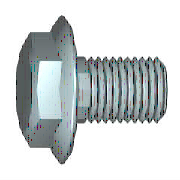
# Autodesk Inventor part: 1_4-20 UNC x 0.625
Saved by Autodesk Inventor 2025.3 (Build 293356030, 356C)
## iProperties
Created: 2024-01-20
Part Number: 1_4-20 UNC x 0.625
Material: Steel, Mild
Description: 1/4"-20 X 5/8" Long Flange Bolt
Document SubType Name: Modeling
Standard: IFI 111
Designer: josh
Standard Revision: 2002
Standards Organization: ANSI
Language: en-US
Size Designation: 1/4-20 UNC x 0.625
Categories: <MemberInstance><Categories><Category DisplayName="Fasteners" InternalName="e4da775c-781d-43d5-af7c-5136215cf5a6" Mnemonic="FSTN"><Category DisplayName="Bolts" InternalName="536e6df0-f778-49ac-b2f2-25c71d2aa0b2" Mnemonic="SCRW"><CategoryParameter DisplayName="Nominal Diameter Designation" InternalName="03caf894-eafd-4c09-a035-916ac084b87b" Mnemonic="nomdiadesig"/><CategoryParameter DisplayName="Nominal Length" InternalName="238ecbaf-3e6c-45dd-aa95-4068c8e0fd02" Mnemonic="nomlen"/><CategoryParameter DisplayName="Thread Designation" InternalName="586d5e89-370a-4089-914f-0110033585c7" Mnemonic="thrdesign"/><CategoryParameter DisplayName="Thread Series Designation" InternalName="87c5849c-b3a5-4c3e-9c9b-2feecef9be86" Mnemonic="thrserdsgn"/><CategoryParameter DisplayName="Nominal Diameter" InternalName="8bbe3f8e-44cf-40a9-a251-3a6edc8168d6" Mnemonic="nomdia"/><CategoryParameter DisplayName="Thread Type" InternalName="b4bbb7bc-d6aa-4c9f-a9a9-4152b9f6fe49" Mnemonic="thrtype"/><CategoryParameter DisplayName="Thread Pitch" InternalName="bb82302e-82d8-4176-8fc1-c5d7bb17d5ad" Mnemonic="pitch1"/><CategoryParameter DisplayName="Threads per Unit" InternalName="bdc6e7d2-ffd0-4d9c-a173-16b95ebb912d" Mnemonic="thrperunit1"/><CategoryParameter DisplayName="Thread Class" InternalName="ebc0d23b-2cc6-4d2a-b376-d52aae53bab6" Mnemonic="thrclss"/><Category DisplayName="Hex Head - Flanged" InternalName="7925b6b6-1575-406f-8bfa-fe006e82b7bc" Mnemonic="FGPLSCREW"><CategoryParameter DisplayName="Width Across Flats" InternalName="448f2cb5-f593-46ea-8e76-5090215a815d" Mnemonic="waflat"/><CategoryParameter DisplayName="Head Height" InternalName="5df4f2f2-b824-4910-9115-49166ccd53b4" Mnemonic="headh"/><CategoryParameter DisplayName="Shank Diameter" InternalName="6799ed14-8456-4cfb-bc01-ee9ecb2cdc2b" Mnemonic="grpdia"/><CategoryParameter DisplayName="Width Across Corners" InternalName="6c4712eb-409b-4c09-a24f-32eb670e2942" Mnemonic="wacor"/><CategoryParameter DisplayName="Type" InternalName="851a99d2-714c-4be1-b4b1-e391fdc059ef" Mnemonic="type"/><CategoryParameter DisplayName="Grip Length" InternalName="a82b65ac-2d41-4fd1-ba9a-aaa8c8b996d2" Mnemonic="grplen"/><CategoryParameter DisplayName="Thread Length" InternalName="f423544c-1850-46c6-9c68-3a3846636699" Mnemonic="thrlen"/></Category></Category></Category><Category DisplayName="DataType" InternalName="23b78d0f-2648-40c6-8793-ca6db495c9e8" Mnemonic="DATATYPE"><CategoryParameter DisplayName="DisplayName" InternalName="05415f3d-3907-474b-a020-eb9d644f4cf3" Mnemonic="DISPLAYNAME"/><CategoryParameter DisplayName="Standard" InternalName="0c0a119c-1e12-4c84-803f-101930972f5e" Mnemonic="STANDARD"/><CategoryParameter DisplayName="Description" InternalName="13903e3d-64b1-4950-80da-f627842ea37f" Mnemonic="DESCRIPTION"/><CategoryParameter DisplayName="Designation" InternalName="2675968c-4ce5-49e0-a4f5-552d29089031" Mnemonic="DESIGNATION"/><CategoryParameter DisplayName="Default Row" InternalName="2af9ec52-faaa-4026-b378-f9fa4afca842" Mnemonic="DEFAULTROW"/><CategoryParameter DisplayName="Folder Name" InternalName="3f06958e-8713-4116-9be7-ed6184ecc97b" Mnemonic="FOLDERNAME"/><CategoryParameter DisplayName="Revision Guid" InternalName="45a75005-10b1-4dfc-8d6d-dfe629f0b93c" Mnemonic="REVISIONGUID"/><CategoryParameter DisplayName="FileName" InternalName="8b46a4cc-9585-4fed-90c3-899f57e09a73" Mnemonic="FILENAME"/><CategoryParameter DisplayName="StdsOrg" InternalName="8f5914e1-4693-403f-8ab5-d37768198c9d" Mnemonic="STDSORG"/><CategoryParameter DisplayName="Family Version" InternalName="914462f6-6e19-4b14-ba84-155b9680b1d0" Mnemonic="FAMILYREVISION"/><CategoryParameter DisplayName="Standard Revision" InternalName="91d5a463-65c2-4fde-b823-3b7fea5e8e17" Mnemonic="STANDARDREVISION"/><CategoryParameter DisplayName="Member Revision" InternalName="a65d44b9-392f-4f4f-857b-e4b3d54996fe" Mnemonic="MEMBERREVISION"/><CategoryParameter DisplayName="ClipFormat" InternalName="bc51e27b-3422-4e78-93ef-cec197ddf230" Mnemonic="CLIPFORMAT"/><CategoryParameter DisplayName="Manufacturer" InternalName="cd6c7a72-a28a-4e50-99a9-2c7f4e13e5ad" Mnemonic="MANUFACTURER"/><CategoryParameter DisplayName="InternalName" InternalName="cf1d0246-76d9-4b4a-8305-fa0409afb5c1" Mnemonic="INTERNALNAME"/><CategoryParameter DisplayName="IsMetric" InternalName="e2385c5b-1ea4-4823-96a8-8de651266ec3" Mnemonic="ISMETRIC"/><Category DisplayName="Part" InternalName="c0e0b642-3bcb-4cc8-9e80-f96d35c4afa4" Mnemonic="PART"><CategoryParameter DisplayName="Part Number" InternalName="016b6077-bfbe-49bd-92c9-d8d59c39c941" Mnemonic="PARTNUMBER"/><CategoryParameter DisplayName="Stock Number" InternalName="4dba7c1c-e26c-444e-836c-b08b433409a8" Mnemonic="STOCKNUMBER"/><CategoryParameter DisplayName="Material Key" InternalName="5c9a8adb-dd2b-4535-b97f-0a94a95fe41f" Mnemonic="MATERIALKEY"/><CategoryParameter DisplayName="Material" InternalName="818a152a-d3c3-49ca-80ee-df7d91421b8e" Mnemonic="MATERIAL"/></Category></Category><Category DisplayName="LegacyMap" InternalName="cd87c42b-3e48-431e-b5c0-1cbeb14dfe77" Mnemonic="LEGACYMAP"><CategoryParameter DisplayName="unique DA member ID" InternalName="0918ad47-427f-4fed-ae26-24c81c58f590" Mnemonic="DACOOKIE"/><CategoryParameter DisplayName="Merge11 ID" InternalName="0ee8fb18-e2ed-4f39-96f6-1f4b5f50aa71" Mnemonic="MERGE11"/><CategoryParameter DisplayName="unique CC member ID" InternalName="5193edd4-b2b0-4ab4-9d54-de900eee34e0" Mnemonic="CCCOOKIE"/><CategoryParameter DisplayName="Split ID" InternalName="72b5c83c-be7f-45c4-ae51-9160ea6deb26" Mnemonic="SPLIT"/><CategoryParameter DisplayName="MemberID" InternalName="8e5e0294-fc51-4c8f-b3d7-003dc5ed94f6" Mnemonic="MEMBERID"/><CategoryParameter DisplayName="CatalogName" InternalName="d99d1e27-aa94-4de2-af4c-c348882a6f4f" Mnemonic="CATALOGNAME"/><CategoryParameter DisplayName="FamilyNumber" InternalName="e705e1f4-09cb-413e-91f9-551b4188271e" Mnemonic="FAMILYNUMBER"/></Category></Categories><FamilyTemplate Id="no0169"><FamilyTemplateParameters><FamilyTemplateParameter ObjectType="kUserParameterObject" ValueType="xs:double" Id="1" ObjectReferenceKey="GUL"/><FamilyTemplateParameter ObjectType="kUserParameterObject" ValueType="xs:double" Id="2" ObjectReferenceKey="SPD"/><FamilyTemplateParameter ObjectType="kUserParameterObject" ValueType="xs:double" Id="3" ObjectReferenceKey="TPU"/><FamilyTemplateParameter ObjectType="kUserParameterObject" ValueType="xs:double" Id="4" ObjectReferenceKey="SD"/><FamilyTemplateParameter ObjectType="kUserParameterObject" ValueType="xs:double" Id="5" ObjectReferenceKey="PHH"/><FamilyTemplateParameter ObjectType="kUserParameterObject" ValueType="xs:double" Id="6" ObjectReferenceKey="PTC"/><FamilyTemplateParameter ObjectType="kUserParameterObject" ValueType="xs:double" Id="7" ObjectReferenceKey="GEL"/><FamilyTemplateParameter ObjectType="kUserParameterObject" ValueType="xs:double" Id="8" ObjectReferenceKey="SW"/><FamilyTemplateParameter ObjectType="kUserParameterObject" ValueType="xs:double" Id="9" ObjectReferenceKey="THREADDIA"/><FamilyTemplateParameter ObjectType="kUserParameterObject" ValueType="xs:double" Id="10" ObjectReferenceKey="SDH"/><FamilyTemplateParameter ObjectType="kUserParameterObject" ValueType="xs:double" Id="11" ObjectReferenceKey="ANG1"/><FamilyTemplateParameter ObjectType="kUserParameterObject" ValueType="xs:double" Id="12" ObjectReferenceKey="TOA"/><FamilyTemplateParameter ObjectType="kUserParameterObject" ValueType="xs:double" Id="13" ObjectReferenceKey="BDM"/><FamilyTemplateParameter ObjectType="kUserParameterObject" ValueType="xs:double" Id="14" ObjectReferenceKey="NLG"/><FamilyTemplateParameter ObjectType="kUserParameterObject" ValueType="xs:double" Id="15" ObjectReferenceKey="KOH"/><FamilyTemplateParameter ObjectType="kUserParameterObject" ValueType="xs:double" Id="16" ObjectReferenceKey="SW0"/><FamilyTemplateParameter ObjectType="kUserParameterObject" ValueType="xs:double" Id="17" ObjectReferenceKey="GD"/><FamilyTemplateParameter ObjectType="kUserParameterObject" ValueType="xs:double" Id="18" ObjectReferenceKey="NND"/><FamilyTemplateParameter ObjectType="kUserParameterObject" ValueType="xs:double" Id="19" ObjectReferenceKey="E0"/><FamilyTemplateParameter ObjectType="kUserParameterObject" ValueType="xs:double" Id="20" ObjectReferenceKey="LADI"/><FamilyTemplateParameter ObjectType="kUserParameterObject" ValueType="xs:double" Id="21" ObjectReferenceKey="GAL"/><FamilyTemplateParameter ObjectType="kUserParameterObject" ValueType="xs:double" Id="22" ObjectReferenceKey="KEWI"/><FamilyTemplateParameter ObjectType="kUserParameterObject" ValueType="xs:double" Id="23" ObjectReferenceKey="SD2"/><FamilyTemplateParameter ObjectType="kUserParameterObject" ValueType="xs:double" Id="24" ObjectReferenceKey="GD1"/><FamilyTemplateParameter ObjectType="kPropertyObject" ValueType="xs:string" Id="100" ObjectReferenceKey="{32853F0F-3444-11d1-9E93-0060B03C1CA6}" SubObjectId="52"/><FamilyTemplateParameter ObjectType="kPropertyObject" ValueType="xs:string" Id="105" ObjectReferenceKey="{32853F0F-3444-11d1-9E93-0060B03C1CA6}" SubObjectId="5"/><FamilyTemplateParameter ObjectType="kPartComponentDefinitionObject" ValueType="xs:string" Id="110" SubObjectId="Material"/><FamilyTemplateParameter ObjectType="kThreadFeatureObject" ValueType="xs:structure" Id="300" ObjectReferenceKey="10020000100000008d070000000000008000000000000000" SubObjectId="ThreadInfo"><FamilyTemplateParameter ObjectType="" ValueType="xs:string" Id="301" SubObjectId="ThreadDesignation"/><FamilyTemplateParameter ObjectType="" ValueType="xs:string" Id="302" SubObjectId="ThreadType"/><FamilyTemplateParameter ObjectType="" ValueType="xs:string" Id="303" SubObjectId="ThreadClass"/></FamilyTemplateParameter></FamilyTemplateParameters></FamilyTemplate><CategoryParameterMap><ParamToTemplateMap><ParamToTemplate CategoryParameter="//CategoryParameter[@InternalName='05415f3d-3907-474b-a020-eb9d644f4cf3']" ConstantValue="Hex Flange Screw - Inch (IFI)"/><ParamToTemplate CategoryParameter="//CategoryParameter[@InternalName='cf1d0246-76d9-4b4a-8305-fa0409afb5c1']" ConstantValue="e9369305-8267-47d2-9425-535ffdf34c16"/><ParamToTemplate CategoryParameter="//CategoryParameter[@InternalName='3f06958e-8713-4116-9be7-ed6184ecc97b']" ConstantValue="IFI 111"/><ParamToTemplate CategoryParameter="//CategoryParameter[@InternalName='914462f6-6e19-4b14-ba84-155b9680b1d0']" ConstantValue="10"/><ParamToTemplate CategoryParameter="//CategoryParameter[@InternalName='bc51e27b-3422-4e78-93ef-cec197ddf230']" ConstantValue="CF_INVENTOR.STDPARTS"/><ParamToTemplate CategoryParameter="//CategoryParameter[@InternalName='e2385c5b-1ea4-4823-96a8-8de651266ec3']" ConstantValue="false"/><ParamToTemplate CategoryParameter="//CategoryParameter[@InternalName='13903e3d-64b1-4950-80da-f627842ea37f']" ConstantValue="Hex Flange Screw - Regular Thread - Inch"/><ParamToTemplate CategoryParameter="//CategoryParameter[@InternalName='8f5914e1-4693-403f-8ab5-d37768198c9d']" ConstantValue="ANSI"/><ParamToTemplate CategoryParameter="//CategoryParameter[@InternalName='0c0a119c-1e12-4c84-803f-101930972f5e']" ConstantValue="IFI 111"/><ParamToTemplate CategoryParameter="//CategoryParameter[@InternalName='cd6c7a72-a28a-4e50-99a9-2c7f4e13e5ad']" TemplateParameter="104"/><ParamToTemplate CategoryParameter="//CategoryParameter[@InternalName='91d5a463-65c2-4fde-b823-3b7fea5e8e17']" ConstantValue="2002"/><ParamToTemplate CategoryParameter="//CategoryParameter[@InternalName='45a75005-10b1-4dfc-8d6d-dfe629f0b93c']" ConstantValue="90fda136-be85-4898-b414-09b1f639c6c8"/><ParamToTemplate CategoryParameter="//CategoryParameter[@InternalName='2af9ec52-faaa-4026-b378-f9fa4afca842']" ConstantValue="10"/><ParamToTemplate CategoryParameter="//CategoryParameter[@InternalName='d99d1e27-aa94-4de2-af4c-c348882a6f4f']" ConstantValue="ANSI"/><ParamToTemplate CategoryParameter="//CategoryParameter[@InternalName='e705e1f4-09cb-413e-91f9-551b4188271e']" ConstantValue="51"/><ParamToTemplate CategoryParameter="//CategoryParameter[@InternalName='8b46a4cc-9585-4fed-90c3-899f57e09a73']" ConstantValue="IFI 111 - 1/4-20 UNC x 0.625"/><ParamToTemplate CategoryParameter="//CategoryParameter[@InternalName='a65d44b9-392f-4f4f-857b-e4b3d54996fe']" ConstantValue="EC67005E-261C-40A7-8008-7B7E2B5E9E01"/><ParamToTemplate CategoryParameter="//CategoryParameter[@InternalName='a82b65ac-2d41-4fd1-ba9a-aaa8c8b996d2']" ConstantValue="0.162"/><ParamToTemplate CategoryParameter="//CategoryParameter[@InternalName='ebc0d23b-2cc6-4d2a-b376-d52aae53bab6']" ConstantValue="2A"/><ParamToTemplate CategoryParameter="//CategoryParameter[@InternalName='87c5849c-b3a5-4c3e-9c9b-2feecef9be86']" ConstantValue="UNC"/><ParamToTemplate CategoryParameter="//CategoryParameter[@InternalName='03caf894-eafd-4c09-a035-916ac084b87b']" ConstantValue="1/4"/><ParamToTemplate CategoryParameter="//CategoryParameter[@InternalName='b4bbb7bc-d6aa-4c9f-a9a9-4152b9f6fe49']" ConstantValue="ANSI Unified Screw Threads"/><ParamToTemplate CategoryParameter="//CategoryParameter[@InternalName='8e5e0294-fc51-4c8f-b3d7-003dc5ed94f6']" ConstantValue="30"/><ParamToTemplate CategoryParameter="//CategoryParameter[@InternalName='6799ed14-8456-4cfb-bc01-ee9ecb2cdc2b']" TemplateParameter="13"/><ParamToTemplate CategoryParameter="//CategoryParameter[@InternalName='2675968c-4ce5-49e0-a4f5-552d29089031']" TemplateParameter="100"/><ParamToTemplate CategoryParameter="//CategoryParameter[@InternalName='6c4712eb-409b-4c09-a24f-32eb670e2942']" TemplateParameter="19"/><ParamToTemplate CategoryParameter="//CategoryParameter[@InternalName='f423544c-1850-46c6-9c68-3a3846636699']" TemplateParameter="7"/><ParamToTemplate CategoryParameter="//CategoryParameter[@InternalName='5df4f2f2-b824-4910-9115-49166ccd53b4']" TemplateParameter="15"/><ParamToTemplate CategoryParameter="//CategoryParameter[@InternalName='818a152a-d3c3-49ca-80ee-df7d91421b8e']" TemplateParameter="110"/><ParamToTemplate CategoryParameter="//CategoryParameter[@InternalName='238ecbaf-3e6c-45dd-aa95-4068c8e0fd02']" TemplateParameter="14"/><ParamToTemplate CategoryParameter="//CategoryParameter[@InternalName='8bbe3f8e-44cf-40a9-a251-3a6edc8168d6']" TemplateParameter="18"/><ParamToTemplate CategoryParameter="//CategoryParameter[@InternalName='016b6077-bfbe-49bd-92c9-d8d59c39c941']" TemplateParameter="105"/><ParamToTemplate CategoryParameter="//CategoryParameter[@InternalName='bb82302e-82d8-4176-8fc1-c5d7bb17d5ad']" TemplateParameter="6"/><ParamToTemplate CategoryParameter="//CategoryParameter[@InternalName='586d5e89-370a-4089-914f-0110033585c7']" TemplateParameter="301"/><ParamToTemplate CategoryParameter="//CategoryParameter[@InternalName='bdc6e7d2-ffd0-4d9c-a173-16b95ebb912d']" TemplateParameter="3"/></ParamToTemplateMap></CategoryParameterMap></MemberInstance>
Density: 7.85 g/cm^3
Appearance: Semi-Polished
Mass: 9.52599 g
Surface Area: 8.24501 cm^2
Volume: 1.2135 cm^3
Flat Length: 0.0
Flat Width: 0.0
Part Area: 0.0
Profile: Purchased Part
IsCustomPart: 1
Author: josh
Autodesk Inventor part; units mm, degrees
ref_plane "YZ Plane" through (0, 0, 0) normal (1, 0, 0) x (0, 1, 0)
ref_plane "XZ Plane" through (0, 0, 0) normal (0, 1, 0) x (-1, 0, 0)
sketch "Sketch1" plane through (0, 0, 0) normal (0, 0, 1) x (1, 0, 0)
  line L0 (-3.2004, 0) -> (-3.2004, 3.8156)
  line L1 (0, 6.096) -> (0, 3.175)
  line L2 (4.1148, 3.175) -> (15.875, 3.175)
  line L3 (15.875, 3.175) -> (15.875, 0)
  line L4 (15.875, 0) -> (-3.2004, 0)
  arc A0 (0, 6.096) -> (-1.9368, 6.5254) centre (-1.016, 6.096) ccw
  line L5 (0, -1.4605) -> (0, 8.7631) projected
  line L6 (-7.0155, 0) -> (19.6901, 0) projected
  line L7 (0, 3.175) -> (0.0001, 3.175)
  line L8 (0.0001, 3.175) -> (0.0001, 3.175)
  line L9 (0.0001, 3.175) -> (2.2098, 3.175)
  line L10 (2.2098, 3.175) -> (4.1148, 3.175)
  line L11 (-3.2004, 3.8156) -> (-1.9368, 6.5254)
  line L12 (0.0001, 3.175) -> (4.1148, 3.175) construction
  line L13 (4.1148, 3.175) -> (4.1148, 0) construction
  dimension "d0" = 1.016
  dimension "d1" = 15.875
  dimension "d2" = 11.7602
  dimension "d3" = 14.224
  dimension "d4" = 6.35
  dimension "d5" = 3.2004
  dimension "d15" = 6.35
  dimension "d16" = 6.35
  dimension "d17" = 0.0001
  dimension "d18" = 1.905
  dimension "d19" = 25
  constraints: 24 end point, 3 collinear, 3 parallel, 2 perpendicular, 2 point on circle, 2 tangent, 1 centre point, 1 point on line, 1 vertical
  measures "d0" radius of A0
  measures "d1" distance between parallel lines of L3 L1
  measures "d2" distance from line of L2.start L3
  measures "d4" diameter of L2 L4
  measures "d5" distance between parallel lines of L1 L0
  measures "d15" diameter of L7 L4
  measures "d16" diameter of L9 L4
  measures "d17" distance from line of L7.end L1
  measures "d18" distance of L2.start L9.end
  measures "d19" angle of L1 L11
revolve "Body" add sketch "Sketch1" angle 360 about axis through (15.875, 0, 0) along (-1, 0, 0)
sketch "Sketch2" plane through (0, 0, 0) normal (1, 0, 0) x (0, 0, -1)
  line L0 (4.7625, 2.7496) -> (4.7625, -2.7496)
  line L1 (4.7625, -2.7496) -> (0, -5.4993)
  line L2 (0, -5.4993) -> (-4.7625, -2.7496)
  line L3 (-4.7625, -2.7496) -> (-4.7625, 2.7496)
  line L4 (-4.7625, 2.7496) -> (0, 5.4993)
  line L5 (0, 5.4993) -> (4.7625, 2.7496)
  point P0 (0, 0)
  point P1 (0, 0)
  dimension "d23" = 9.525
  constraints: 12 end point, 1 coincident, 1 vertical, 11 other
  measures "d23" distance between parallel lines of L3 L0
extrude "Head" add sketch "Sketch2" against normal blind 7.112
sketch "Sketch3" plane through (0, 0, 0) normal (0, 0, 1) x (1, 0, 0)
  line L0 (-7.112, 4.7625) -> (-7.112, 5.4993)
  line L1 (-7.112, 5.4993) -> (-6.6866, 5.4993)
  line L2 (-6.6866, 5.4993) -> (-7.112, 4.7625)
  line L3 (-8.0513, 0) -> (-1.476, 0) projected
  line L4 (-7.112, 5.4993) -> (-7.112, 2.7496) projected
  line L5 (-2.4153, 5.4993) -> (-7.112, 5.4993) projected
  point P0 (-7.112, 2.7496)
  dimension "d8" = 30
  dimension "d22" = 9.525
  constraints: 6 end point, 2 collinear, 1 perpendicular
  measures "d8" angle of L2 L0
  measures "d22" diameter of L0.start L3
revolve "Chamfer1" cut sketch "Sketch3" angle 360 about axis through (-10, 0, 0) along (1, 0, 0)
thread "Thread" size "1/4-20 UNC" class "2A" standard "ANSI Unified Screw Threads" length 11.7602
chamfer "Chamfer2" distance 0.7791 distance2 0.7791 1 edges at (15.875, -3.175, 0) measured on face at (15.875, 0.0371, -1.7957)
ref_plane "Work Plane1" through (10.95, 0, 0) normal (0, 0, -1) x (1, 0, 0)
equation "\"d23\" = SW"
equation "\"d6\" = KOH"
equation "\"d10\" = GEL"
equation "\"d13\" = -0.5 * SPD + 0.5 * GD"
equation "\"d14\" = GUL"
equation "\"d0\" = PHH"
equation "\"d1\" = NLG"
equation "\"d2\" = GEL"
equation "\"d3\" = LADI"
equation "\"d4\" = GD"
equation "\"d5\" = 0.45 * KOH"
equation "\"d15\" = SD2"
equation "\"d16\" = BDM"
equation "\"d18\" = GAL"
equation "\"d19\" = KEWI"
equation "\"d8\" = ANG1"
equation "\"d22\" = SW0"
equation "\"NLG\" = 15.875"
equation "\"GD\" = NND"
equation "\"BDM\" = NND"
equation "\"KOH\" = 7.112"
equation "\"GEL\" = 11.7602"
equation "\"LADI\" = 14.224"
equation "\"SW\" = 9.525"
equation "\"PHH\" = 1.016"
equation "\"SW0\" = SW"
equation "\"SPD\" = 4.79184"
equation "\"SD2\" = NND"
equation "\"SD\" = 0"
equation "\"ANG1\" = 30deg"
equation "\"KEWI\" = 25deg"
equation "\"GAL\" = 1.905"
equation "\"GUL\" = 0.77908"
equation "\"THREADDIA\" = 6.35"
equation "\"SDH\" = SW"
equation "\"TOA\" = 30deg"
equation "\"NND\" = 6.35"
equation "\"E0\" = 1.155 * SW"
equation "\"GD1\" = 4.79184"
body "Solid1"
